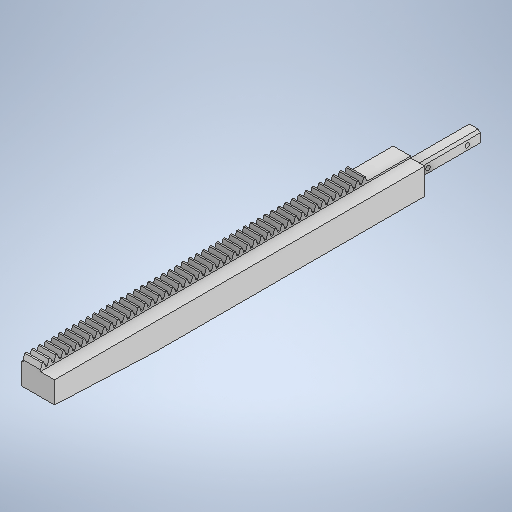
# Autodesk Inventor part: cremaillere
Saved by Autodesk Inventor 2025.2 (Build 292293000, 293)
## iProperties
Created: 2025-03-30
Part Number: cremaillere
Material: Générique
Document SubType Name: Modeling
Designer: enezl
Density: 1 g/cm^3
Appearance: Par défaut
Author: enezl
Autodesk Inventor part; units mm, degrees
ref_plane "YZ Plane" through (0, 0, 0) normal (1, 0, 0) x (0, 1, 0)
ref_plane "XZ Plane" through (0, 0, 0) normal (0, 1, 0) x (-1, 0, 0)
sketch "dent" plane through (0, 0, 0) normal (0, 0, 1) x (1, 0, 0)
  line L0 (3.4049, 12.8641) -> (5.6549, 12.0451)
  line L1 (5.6549, 12.0451) -> (5.6549, 11.2941)
  line L2 (5.6549, 11.2941) -> (3.4049, 10.4751)
  line L3 (3.4049, 10.4751) -> (3.4049, 9.7241)
  point P0 (4.4433, 11.2784)
  dimension "d0" = 2.25
  dimension "d1" = 110
  dimension "d2" = 40
  dimension "d3" = 3.14
  measures "d3" distance of point (3.405, 9.724) point (3.405, 12.864)
sketch "Esquisse1" plane through (0, 0, 0) normal (1, 0, 0) x (0, 1, 0)
  line L0 (12.75, 135) -> (12.75, -15) construction
  line L1 (12.75, 135) -> (2, 135)
  line L2 (0, 135) -> (0, -135) construction
  line L3 (0, -135) -> (12.75, -135) construction
  line L4 (12.75, -15.72) -> (12.75, -35)
  line L5 (2, 135) -> (0, 89.1925)
  line L6 (2, 135) -> (0, 135) construction
  line L7 (0, 89.1925) -> (0, -35)
  line L8 (0, -35) -> (12.75, -35)
  line L9 (12.75, -35) -> (12.75, -135) construction
  line L10 (0, -35) -> (0, -135) construction
  line L11 (12.75, 135) -> (15, 134.1811)
  line L12 (15, 134.1811) -> (15, 133.43)
  line L13 (15, 133.43) -> (12.75, 132.6111)
  line L14 (12.75, 132.6111) -> (12.75, 131.86)
  line L15 (12.75, 131.86) -> (15, 131.0411)
  line L16 (15, 131.0411) -> (15, 130.29)
  line L17 (15, 130.29) -> (12.75, 129.4711)
  line L18 (12.75, 129.4711) -> (12.75, 128.72)
  line L19 (12.75, 128.72) -> (15, 127.9011)
  line L20 (15, 127.9011) -> (15, 127.15)
  line L21 (15, 127.15) -> (12.75, 126.3311)
  line L22 (12.75, 126.3311) -> (12.75, 125.58)
  line L23 (12.75, 125.58) -> (15, 124.7611)
  line L24 (15, 124.7611) -> (15, 124.01)
  line L25 (15, 124.01) -> (12.75, 123.1911)
  line L26 (12.75, 123.1911) -> (12.75, 122.44)
  line L27 (12.75, 122.44) -> (15, 121.6211)
  line L28 (15, 121.6211) -> (15, 120.87)
  line L29 (15, 120.87) -> (12.75, 120.0511)
  line L30 (12.75, 120.0511) -> (12.75, 119.3)
  line L31 (12.75, 119.3) -> (15, 118.4811)
  line L32 (15, 118.4811) -> (15, 117.73)
  line L33 (15, 117.73) -> (12.75, 116.9111)
  line L34 (12.75, 116.9111) -> (12.75, 116.16)
  line L35 (12.75, 116.16) -> (15, 115.3411)
  line L36 (15, 115.3411) -> (15, 114.59)
  line L37 (15, 114.59) -> (12.75, 113.7711)
  line L38 (12.75, 113.7711) -> (12.75, 113.02)
  line L39 (12.75, 113.02) -> (15, 112.2011)
  line L40 (15, 112.2011) -> (15, 111.45)
  line L41 (15, 111.45) -> (12.75, 110.6311)
  line L42 (12.75, 110.6311) -> (12.75, 109.88)
  line L43 (12.75, 109.88) -> (15, 109.0611)
  line L44 (15, 109.0611) -> (15, 108.31)
  line L45 (15, 108.31) -> (12.75, 107.4911)
  line L46 (12.75, 107.4911) -> (12.75, 106.74)
  line L47 (12.75, 106.74) -> (15, 105.9211)
  line L48 (15, 105.9211) -> (15, 105.17)
  line L49 (15, 105.17) -> (12.75, 104.3511)
  line L50 (12.75, 104.3511) -> (12.75, 103.6)
  line L51 (12.75, 103.6) -> (15, 102.7811)
  line L52 (15, 102.7811) -> (15, 102.03)
  line L53 (15, 102.03) -> (12.75, 101.2111)
  line L54 (12.75, 101.2111) -> (12.75, 100.46)
  line L55 (12.75, 100.46) -> (15, 99.6411)
  line L56 (15, 99.6411) -> (15, 98.89)
  line L57 (15, 98.89) -> (12.75, 98.0711)
  line L58 (12.75, 98.0711) -> (12.75, 97.32)
  line L59 (12.75, 97.32) -> (15, 96.5011)
  line L60 (15, 96.5011) -> (15, 95.75)
  line L61 (15, 95.75) -> (12.75, 94.9311)
  line L62 (12.75, 94.9311) -> (12.75, 94.18)
  line L63 (12.75, 94.18) -> (15, 93.3611)
  line L64 (15, 93.3611) -> (15, 92.61)
  line L65 (15, 92.61) -> (12.75, 91.7911)
  line L66 (12.75, 91.7911) -> (12.75, 91.04)
  line L67 (12.75, 91.04) -> (15, 90.2211)
  line L68 (15, 90.2211) -> (15, 89.47)
  line L69 (15, 89.47) -> (12.75, 88.6511)
  line L70 (12.75, 88.6511) -> (12.75, 87.9)
  line L71 (12.75, 87.9) -> (15, 87.0811)
  line L72 (15, 87.0811) -> (15, 86.33)
  line L73 (15, 86.33) -> (12.75, 85.5111)
  line L74 (12.75, 85.5111) -> (12.75, 84.76)
  line L75 (12.75, 84.76) -> (15, 83.9411)
  line L76 (15, 83.9411) -> (15, 83.19)
  line L77 (15, 83.19) -> (12.75, 82.3711)
  line L78 (12.75, 82.3711) -> (12.75, 81.62)
  line L79 (12.75, 81.62) -> (15, 80.8011)
  line L80 (15, 80.8011) -> (15, 80.05)
  line L81 (15, 80.05) -> (12.75, 79.2311)
  line L82 (12.75, 79.2311) -> (12.75, 78.48)
  line L83 (12.75, 78.48) -> (15, 77.6611)
  line L84 (15, 77.6611) -> (15, 76.91)
  line L85 (15, 76.91) -> (12.75, 76.0911)
  line L86 (12.75, 76.0911) -> (12.75, 75.34)
  line L87 (12.75, 75.34) -> (15, 74.5211)
  line L88 (15, 74.5211) -> (15, 73.77)
  line L89 (15, 73.77) -> (12.75, 72.9511)
  line L90 (12.75, 72.9511) -> (12.75, 72.2)
  line L91 (12.75, 72.2) -> (15, 71.3811)
  line L92 (15, 71.3811) -> (15, 70.63)
  line L93 (15, 70.63) -> (12.75, 69.8111)
  line L94 (12.75, 69.8111) -> (12.75, 69.06)
  line L95 (12.75, 69.06) -> (15, 68.2411)
  line L96 (15, 68.2411) -> (15, 67.49)
  line L97 (15, 67.49) -> (12.75, 66.6711)
  line L98 (12.75, 66.6711) -> (12.75, 65.92)
  line L99 (12.75, 65.92) -> (15, 65.1011)
  line L100 (15, 65.1011) -> (15, 64.35)
  line L101 (15, 64.35) -> (12.75, 63.5311)
  line L102 (12.75, 63.5311) -> (12.75, 62.78)
  line L103 (12.75, 62.78) -> (15, 61.9611)
  line L104 (15, 61.9611) -> (15, 61.21)
  line L105 (15, 61.21) -> (12.75, 60.3911)
  line L106 (12.75, 60.3911) -> (12.75, 59.64)
  line L107 (12.75, 59.64) -> (15, 58.8211)
  line L108 (15, 58.8211) -> (15, 58.07)
  line L109 (15, 58.07) -> (12.75, 57.2511)
  line L110 (12.75, 57.2511) -> (12.75, 56.5)
  line L111 (12.75, 56.5) -> (15, 55.6811)
  line L112 (15, 55.6811) -> (15, 54.93)
  line L113 (15, 54.93) -> (12.75, 54.1111)
  line L114 (12.75, 54.1111) -> (12.75, 53.36)
  line L115 (12.75, 53.36) -> (15, 52.5411)
  line L116 (15, 52.5411) -> (15, 51.79)
  line L117 (15, 51.79) -> (12.75, 50.9711)
  line L118 (12.75, 50.9711) -> (12.75, 50.22)
  line L119 (12.75, 50.22) -> (15, 49.4011)
  line L120 (15, 49.4011) -> (15, 48.65)
  line L121 (15, 48.65) -> (12.75, 47.8311)
  line L122 (12.75, 47.8311) -> (12.75, 47.08)
  line L123 (12.75, 47.08) -> (15, 46.2611)
  line L124 (15, 46.2611) -> (15, 45.51)
  line L125 (15, 45.51) -> (12.75, 44.6911)
  line L126 (12.75, 44.6911) -> (12.75, 43.94)
  line L127 (12.75, 43.94) -> (15, 43.1211)
  line L128 (15, 43.1211) -> (15, 42.37)
  line L129 (15, 42.37) -> (12.75, 41.5511)
  line L130 (12.75, 41.5511) -> (12.75, 40.8)
  line L131 (12.75, 40.8) -> (15, 39.9811)
  line L132 (15, 39.9811) -> (15, 39.23)
  line L133 (15, 39.23) -> (12.75, 38.4111)
  line L134 (12.75, 38.4111) -> (12.75, 37.66)
  line L135 (12.75, 37.66) -> (15, 36.8411)
  line L136 (15, 36.8411) -> (15, 36.09)
  line L137 (15, 36.09) -> (12.75, 35.2711)
  line L138 (12.75, 35.2711) -> (12.75, 34.52)
  line L139 (12.75, 34.52) -> (15, 33.7011)
  line L140 (15, 33.7011) -> (15, 32.95)
  line L141 (15, 32.95) -> (12.75, 32.1311)
  line L142 (12.75, 32.1311) -> (12.75, 31.38)
  line L143 (12.75, 31.38) -> (15, 30.5611)
  line L144 (15, 30.5611) -> (15, 29.81)
  line L145 (15, 29.81) -> (12.75, 28.9911)
  line L146 (12.75, 28.9911) -> (12.75, 28.24)
  line L147 (12.75, 28.24) -> (15, 27.4211)
  line L148 (15, 27.4211) -> (15, 26.67)
  line L149 (15, 26.67) -> (12.75, 25.8511)
  line L150 (12.75, 25.8511) -> (12.75, 25.1)
  line L151 (12.75, 25.1) -> (15, 24.2811)
  line L152 (15, 24.2811) -> (15, 23.53)
  line L153 (15, 23.53) -> (12.75, 22.7111)
  line L154 (12.75, 22.7111) -> (12.75, 21.96)
  line L155 (12.75, 21.96) -> (15, 21.1411)
  line L156 (15, 21.1411) -> (15, 20.39)
  line L157 (15, 20.39) -> (12.75, 19.5711)
  line L158 (12.75, 19.5711) -> (12.75, 18.82)
  line L159 (12.75, 18.82) -> (15, 18.0011)
  line L160 (15, 18.0011) -> (15, 17.25)
  line L161 (15, 17.25) -> (12.75, 16.4311)
  line L162 (12.75, 16.4311) -> (12.75, 15.68)
  line L163 (12.75, 15.68) -> (15, 14.8611)
  line L164 (15, 14.8611) -> (15, 14.11)
  line L165 (15, 14.11) -> (12.75, 13.2911)
  line L166 (12.75, 13.2911) -> (12.75, 12.54)
  line L167 (12.75, 12.54) -> (15, 11.7211)
  line L168 (15, 11.7211) -> (15, 10.97)
  line L169 (15, 10.97) -> (12.75, 10.1511)
  line L170 (12.75, 10.1511) -> (12.75, 9.4)
  line L171 (12.75, 9.4) -> (15, 8.5811)
  line L172 (15, 8.5811) -> (15, 7.83)
  line L173 (15, 7.83) -> (12.75, 7.0111)
  line L174 (12.75, 7.0111) -> (12.75, 6.26)
  line L175 (12.75, 6.26) -> (15, 5.4411)
  line L176 (15, 5.4411) -> (15, 4.69)
  line L177 (15, 4.69) -> (12.75, 3.8711)
  line L178 (12.75, 3.8711) -> (12.75, 3.12)
  line L179 (12.75, 3.12) -> (15, 2.3011)
  line L180 (15, 2.3011) -> (15, 1.55)
  line L181 (15, 1.55) -> (12.75, 0.7311)
  line L182 (12.75, 0.7311) -> (12.75, -0.02)
  line L183 (12.75, -0.02) -> (15, -0.8389)
  line L184 (15, -0.8389) -> (15, -1.59)
  line L185 (15, -1.59) -> (12.75, -2.4089)
  line L186 (12.75, -2.4089) -> (12.75, -3.16)
  line L187 (12.75, -3.16) -> (15, -3.9789)
  line L188 (15, -3.9789) -> (15, -4.73)
  line L189 (15, -4.73) -> (12.75, -5.5489)
  line L190 (12.75, -5.5489) -> (12.75, -6.3)
  line L191 (12.75, -6.3) -> (15, -7.1189)
  line L192 (15, -7.1189) -> (15, -7.87)
  line L193 (15, -7.87) -> (12.75, -8.6889)
  line L194 (12.75, -8.6889) -> (12.75, -9.44)
  line L195 (12.75, -9.44) -> (15, -10.2589)
  line L196 (15, -10.2589) -> (15, -11.01)
  line L197 (15, -11.01) -> (12.75, -11.8289)
  line L198 (12.75, -11.8289) -> (12.75, -12.58)
  line L199 (12.75, -12.58) -> (15, -13.3989)
  line L200 (15, -13.3989) -> (15, -14.15)
  line L201 (15, -14.15) -> (12.75, -14.9689)
  line L202 (12.75, -14.9689) -> (12.75, -15.72)
  point P0 (0, 0)
  point P1 (0, 0)
  point P2 (12.75, -12.58)
  point P3 (12.75, -6.3)
  point P4 (12.75, -3.16)
  point P5 (12.75, -0.02)
  point P6 (12.75, 3.12)
  point P7 (12.75, 9.4)
  point P8 (12.75, 12.54)
  point P9 (12.75, 18.82)
  point P10 (12.75, 21.96)
  point P11 (12.75, 25.1)
  point P12 (12.75, 28.24)
  point P13 (12.75, 31.38)
  point P14 (12.75, 34.52)
  point P15 (12.75, 37.66)
  point P16 (12.75, 40.8)
  point P17 (12.75, 47.08)
  point P18 (12.75, 50.22)
  point P19 (12.75, 53.36)
  point P20 (12.75, 56.5)
  point P21 (12.75, 59.64)
  point P22 (12.75, 62.78)
  point P23 (12.75, 65.92)
  point P24 (12.75, 69.06)
  point P25 (12.75, 78.48)
  point P26 (12.75, 81.62)
  point P27 (12.75, 84.76)
  point P28 (12.75, 87.9)
  point P29 (12.75, 91.04)
  point P30 (12.75, 94.18)
  point P31 (12.75, 106.74)
  point P32 (12.75, 113.02)
  point P33 (12.75, 119.3)
  point P34 (12.75, 125.58)
  point P35 (12.75, 131.86)
  dimension "d7" = 3.14
  dimension "d4" = 150
  dimension "d12" = 15
  dimension "d13" = 270
  dimension "d14" = 2.5
  dimension "d15" = 2
  dimension "d42" = 170
  constraints: 51 vertical, 22 end point, 4 perpendicular, 2 collinear, 2 horizontal, 1 coincident, 1 midpoint, 1 point on line, 2 other
  measures "d4" distance of L0.start L0.end
  measures "d13" distance of L2.start L2.end
  measures "d14" angle of L2 L5
  measures "d15" distance of L1.end L2.start
  measures "d42" distance between parallel lines of L1 L8
extrude "Extrusion1" add sketch "Esquisse1" along normal blind 8
sketch "Esquisse2" plane through (8, 0, 0) normal (1, 0, 0) x (0, 0, -1)
  line L0 (-135, 2) -> (-89.1925, 0) projected
  line L1 (-135, 12.75) -> (-135, 2) construction
  line L2 (-89.1925, 0) -> (35, 0) projected
  line L3 (-135, 12.75) -> (-135, 2) construction
  line L4 (-135, 12) -> (35, 12)
  line L5 (-135, 12) -> (-135, 2)
  line L6 (115, 12) -> (115, 12.75) construction
  line L7 (35, 12.75) -> (14.9689, 12.75) construction
  line L8 (35, 0) -> (35, 12)
  point P0 (0, 0)
  dimension "d37" = 12
  constraints: 8 end point, 2 point on line, 1 collinear, 1 horizontal, 1 perpendicular, 1 vertical
  measures "d37" distance between parallel lines of L2 L4
extrude "Extrusion2" add sketch "Esquisse2" along normal blind 6.5 and the other way blind 8.5
ref_plane "Plan de construction1" through (7, 0, 0) normal (-1, 0, 0) x (0, 0, 1)
sketch "Esquisse5" plane through (7, 0, 0) normal (-1, 0, 0) x (0, 0, 1)
  line L0 (-65, 9) -> (-35, 9)
  line L1 (-35, 9) -> (-35, 3)
  line L2 (-35, 3) -> (-65, 3)
  line L3 (-65, 3) -> (-65, 9)
  line L4 (-65, 9) -> (-35, 3) construction
  line L5 (-35, 9) -> (-65, 3) construction
  line L6 (-35, 0) -> (-35, 12) construction
  point P0 (0, 0)
  point P1 (-50, 6)
  point P2 (-35, 6)
  dimension "d43" = 6
  dimension "d44" = 30
  constraints: 12 end point, 4 midpoint, 2 parallel, 1 horizontal, 1 perpendicular
  measures "d43" distance of L0.end L1.end
  measures "d44" distance of L1.end L2.end
extrude "Extrusion5" add sketch "Esquisse5" along normal mid plane 6
chamfer "Chanfrein1" distance 1 angle 45 4 edges at (10, 9, -50) (4, 9, -50) (10, 3, -50) (4, 3, -50)
sketch "Esquisse6" plane through (10, 0, 0) normal (1, 0, 0) x (0, 0, -1)
  line L0 (65, 4) -> (35, 4) construction
  line L1 (65, 4) -> (65, 8) construction
  line L2 (35, 8) -> (65, 8) construction
  line L3 (35, 4) -> (35, 8) construction
  line L4 (35, 6) -> (65, 6) construction
  line L5 (65, 4) -> (65, 8) projected
  line L6 (41, 6) -> (59, 6) construction
  point P0 (0, 0)
  point P1 (50, 6)
  dimension "d50" = 18
  constraints: 5 midpoint, 4 end point, 2 point on line, 1 collinear
  measures "d50" distance of L6.end L6.start
hole "Perçage2" at (10, 6, -41) at (10, 6, -59) direction (-1, 0, 0) diameter 2.1 end through all
